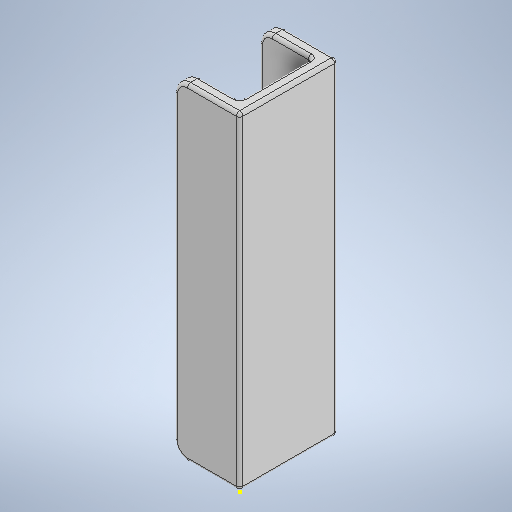
# Autodesk Inventor part: Соединитель
Saved by Autodesk Inventor 2025 (Build 290162000, 162)
## iProperties
Created: 2025-05-20
Part Number: Соединитель
Material: Типовые
Document SubType Name: Modeling
Designer: vinogradov
Density: 1 g/cm^3
Appearance: По умолчанию
Author: vinogradov
Autodesk Inventor part; units mm, degrees
ref_plane "YZ Plane" through (0, 0, 0) normal (1, 0, 0) x (0, 1, 0)
ref_plane "XZ Plane" through (0, 0, 0) normal (0, 1, 0) x (-1, 0, 0)
ref_plane "XY Plane" through (0, 0, 0) normal (0, 0, 1) x (1, 0, 0)
sketch "Эскиз1" plane through (0, 0, 0) normal (0, 1, 0) x (-1, 0, 0)
  point P0 (0, 0)
sketch "Эскиз2" plane through (0, 0, 0) normal (0, 1, 0) x (-1, 0, 0)
  line L0 (0, 0) -> (10, 0)
  line L1 (10, 0) -> (10, -2)
  line L2 (10, -2) -> (2, -2)
  line L3 (2, -2) -> (2, -13)
  line L4 (2, -13) -> (10, -13)
  line L5 (10, -13) -> (10, -15)
  line L6 (10, -15) -> (0, -15)
  line L7 (0, -15) -> (0, 0)
  dimension "d0" = 10
  dimension "d1" = 2
  dimension "d3" = 11
  dimension "d4" = 2
  dimension "d5" = 2
  constraints: 16 end point, 6 perpendicular, 2 point on line, 1 horizontal
  measures "d0" distance of L0.start L0.end
  measures "d1" distance of L0.end L1.end
  measures "d3" distance of L2.end L3.end
  measures "d4" distance of L4.end L5.end
  measures "d5" distance between parallel lines of L7 L3
extrude "Выдавливание1" add sketch "Эскиз2" along normal blind 50
fillet "Сопряжение1" radius 2 4 edges at (-10, 50, -14) (-10, 50, -1) (-10, 0, -14) (-10, 0, -1)
fillet "Сопряжение2" radius 0.5 28 edges at (0, 25, -15) (-9.4142, 49.4142, -15) (-10, 25, -15) (-9.4142, 0.5858, -15) (-4, 0, -15) (-4, 50, -15) (-9.4142, 49.4142, -13) (-10, 25, -13) (-9.4142, 0.5858, -13) (-5, 0, -13) (-5, 50, -13) (-2, 50, -7.5) (0, 50, -7.5) (-9.4142, 49.4142, 0) (-10, 25, 0) (-9.4142, 0.5858, 0) (-4, 0, 0) (-4, 50, 0) (-9.4142, 49.4142, -2) (-10, 25, -2) (-9.4142, 0.5858, -2) (-5, 0, -2) (-5, 50, -2) (-2, 25, -2) (-2, 0, -7.5) (0, 0, -7.5) (-2, 25, -13) (0, 25, 0)
